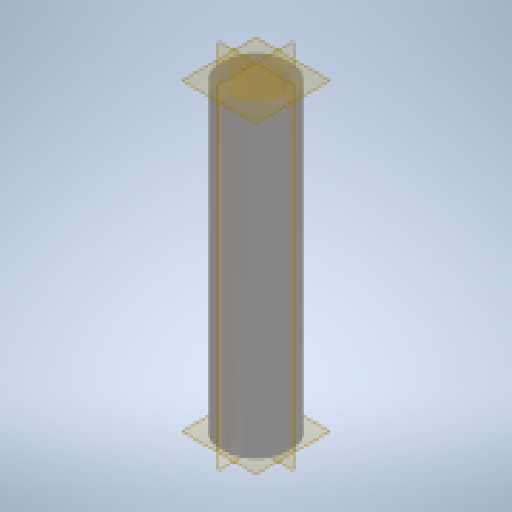
# Autodesk Inventor part: Z1
Saved by Autodesk Inventor 2025.2 (Build 292293000, 293)
## iProperties
Created: 2025-03-23
Part Number: Z1
Material: Steel, Alloy
Document SubType Name: Modeling
Designer: MSIGAMING
Mass: 95620.3 g
Surface Area: 10170.9 cm^2
Volume: 12370 cm^3
Density: 7.73 g/cm^3
Appearance: Semi-Polished
Author: MSIGAMING
Autodesk Inventor part; units mm, degrees
sketch "Sketch1" plane through (0, 0, 0) normal (0, 1, 0) x (-1, 0, 0)
  circle A0 centre (0, 0) radius 100
  circle A1 centre (0, 0) radius 75
  dimension "d0" = 200
  dimension "d3" = 150
  constraints: 2 centre point, 2 coincident
  measures "d0" diameter of A0
  measures "d3" diameter of A1
extrude "Extrusion1" add sketch "Sketch1" along normal blind 900
ref_plane "Work Plane1" through (0, 900, 0) normal (0, 1, 0) x (1, 0, 0)
body "Solid1"
